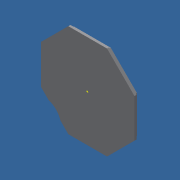
# Autodesk Inventor part: Oktagon_Deckel
Saved by Autodesk Inventor 2018.2 (Build 222227000, 227)
## iProperties
Created: 2018-10-01
Part Number: Oktagon_Deckel
Material: geeigneten Werkstoff auswählen !
Document SubType Name: Modeling
Designer: N.Grubert
Density: 0.001 g/cm^3
Appearance: Vorgabe
Fläche: 0 cm²
Gewicht: 0 g
Dateiname: P:\INVENTOR\Inventor 2018\Templates\ILT\Norm.ipt
Bez_eng: bolt
Bez_french: boulon
Author: N.Grubert
Autodesk Inventor part; units mm, degrees
ref_plane "YZ Plane" through (0, 0, 0) normal (1, 0, 0) x (0, 1, 0)
ref_plane "XZ Plane" through (0, 0, 0) normal (0, 1, 0) x (-1, 0, 0)
ref_plane "XY Plane" through (0, 0, 0) normal (0, 0, 1) x (1, 0, 0)
sketch "Skizze4" plane through (0, 0, 0) normal (0, 1, 0) x (-1, 0, 0)
  line L0 (22.7817, 55) -> (55, 22.7817)
  line L1 (55, 22.7817) -> (55, -22.7817)
  line L2 (55, -22.7817) -> (22.7817, -55)
  line L3 (22.7817, -55) -> (-22.7817, -55)
  line L4 (-22.7817, -55) -> (-55, -22.7817)
  line L5 (-55, -22.7817) -> (-55, 22.7817)
  line L6 (-55, 22.7817) -> (-22.7817, 55)
  line L7 (-22.7817, 55) -> (22.7817, 55)
  line L8 (0, -77) -> (0, 77) construction
  line L9 (77, 0) -> (-77, 0) construction
  point P0 (0, 0)
  point P1 (0, 0)
  dimension "d4" = 110
  constraints: 16 end point, 1 coincident, 18 other
  measures "d4" distance between parallel lines of L3 L7
extrude "Extrusion2" add sketch "Skizze4" along normal blind 2.5
sketch "Skizze5" plane through (0, 2.5, 0) normal (0, 1, 0) x (1, 0, 0)
  line L0 (21.7462, 52.5) -> (-21.7462, 52.5) projected
  line L1 (-21.7462, 52.5) -> (-52.5, 21.7462) projected
  line L2 (-52.5, 21.7462) -> (-52.5, -21.7462) projected
  line L3 (-52.5, -21.7462) -> (-21.7462, -52.5) projected
  line L4 (-21.7462, -52.5) -> (21.7462, -52.5) projected
  line L5 (21.7462, -52.5) -> (52.5, -21.7462) projected
  line L6 (52.5, -21.7462) -> (52.5, 21.7462) projected
  line L7 (52.5, 21.7462) -> (21.7462, 52.5) projected
  line L8 (22.7817, 55) -> (55, 22.7817) projected
  line L9 (55, 22.7817) -> (55, -22.7817) projected
  line L10 (55, -22.7817) -> (22.7817, -55) projected
  line L11 (22.7817, -55) -> (-22.7817, -55) projected
  line L12 (-22.7817, -55) -> (-55, -22.7817) projected
  line L13 (-55, -22.7817) -> (-55, 22.7817) projected
  line L14 (-55, 22.7817) -> (-22.7817, 55) projected
  line L15 (-22.7817, 55) -> (22.7817, 55) projected
  line L16 (-50, 20.7107) -> (-20.7107, 50)
  line L17 (-20.7107, 50) -> (20.7107, 50)
  line L18 (20.7107, 50) -> (50, 20.7107)
  line L19 (50, 20.7107) -> (50, -20.7107)
  line L20 (50, -20.7107) -> (20.7107, -50)
  line L21 (20.7107, -50) -> (-20.7107, -50)
  line L22 (-20.7107, -50) -> (-50, -20.7107)
  line L23 (-50, -20.7107) -> (-50, 20.7107)
  point P0 (0, 0)
  dimension "d7" = 2.5
  constraints: 16 end point, 7 other
  measures "d7" distance between parallel lines of L0 L17
extrude "Extrusion3" add sketch "Skizze5" along normal blind 3 contours L7 L6 L5 L4 L3 L2 L1 L0
sketch "Skizze7" plane through (0, 0, 0) normal (0, -1, 0) x (1, 0, 0)
  line L0 (-22.7817, 55) -> (-55, 22.7817) construction
  line L1 (-55, 22.7817) -> (-55, -22.7817) construction
  line L2 (-55, -22.7817) -> (-22.7817, -55) construction
  line L3 (-22.7817, -55) -> (22.7817, -55) construction
  line L4 (22.7817, -55) -> (55, -22.7817) construction
  line L5 (55, -22.7817) -> (55, 22.7817) construction
  line L6 (55, 22.7817) -> (22.7817, 55) construction
  line L7 (22.7817, 55) -> (-22.7817, 55) construction
  line L8 (-55, 22.7817) -> (-55, -22.7817) projected
  arc A0 (-55, 9.6687) -> (-55, -9.9272) centre (-45, -0.1293) ccw
  point P0 (0, 0)
  dimension "d15" = 14
  dimension "d16" = 10
  constraints: 2 point on circle, 2 point on line, 1 centre point
  measures "d15" radius of A0
  measures "d16" distance from line of L1 A0.centre
extrude "Extrusion5" add sketch "Skizze7" against normal up to surface (2.5 mm away)
